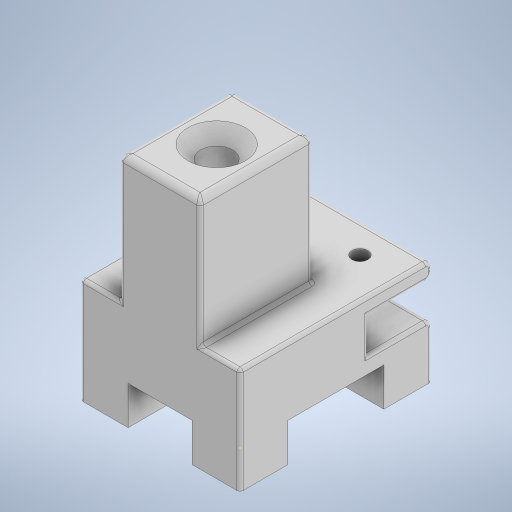
# Autodesk Inventor part: PortaHerramienta1
Saved by Autodesk Inventor 2024 (Build 280153000, 153)
## iProperties
Created: 2023-11-06
Part Number: PortaHerramienta1
Material: Generic
Document SubType Name: Modeling
Designer: Juan_Daleman
Density: 1 g/cm^3
Appearance: Default
Author: Juan_Daleman
Autodesk Inventor part; units mm, degrees
ref_plane "YZ Plane" through (0, 0, 0) normal (1, 0, 0) x (0, 1, 0)
ref_plane "XZ Plane" through (0, 0, 0) normal (0, 1, 0) x (-1, 0, 0)
ref_plane "XY Plane" through (0, 0, 0) normal (0, 0, 1) x (1, 0, 0)
sketch "Sketch1" plane through (0, 0, 0) normal (0, 1, 0) x (-1, 0, 0)
  line L0 (0, 0) -> (50, 0)
  line L1 (50, 0) -> (50, -60)
  line L2 (50, -60) -> (0, -60)
  line L3 (0, -60) -> (0, 0)
  dimension "d0" = 50
  dimension "d1" = 60
  constraints: 8 end point, 2 parallel, 1 horizontal, 1 perpendicular
  measures "d0" distance of L1.end L2.end
  measures "d1" distance of L0.end L1.end
extrude "Extrusion1" add sketch "Sketch1" along normal blind 5
sketch "Sketch2" plane through (0, 5, 0) normal (0, 1, 0) x (1, 0, 0)
  line L0 (-50, 0) -> (0, 0) projected
  line L1 (-50, 60) -> (-50, 0) projected
  line L2 (0, 0) -> (-50, 0)
  line L3 (-50, 0) -> (-50, 40)
  line L4 (-50, 40) -> (0, 40)
  line L5 (0, 40) -> (0, 0)
  dimension "d4" = 40
  constraints: 8 end point, 2 parallel, 1 horizontal, 1 perpendicular, 1 point on line
  measures "d4" distance of L2.end L3.end
extrude "Extrusion2" add sketch "Sketch2" along normal blind 11
sketch "Sketch3" plane through (0, 16, 0) normal (0, 1, 0) x (1, 0, 0)
  line L0 (0, 0) -> (-50, 0)
  line L1 (-50, 0) -> (-50, 60)
  line L2 (-50, 60) -> (0, 60)
  line L3 (0, 60) -> (0, 0)
  constraints: 8 end point, 2 parallel, 1 horizontal, 1 perpendicular
extrude "Extrusion3" add sketch "Sketch3" along normal blind 5
sketch "Sketch4" plane through (0, 21, 0) normal (0, 1, 0) x (1, 0, 0)
  line L0 (0, 0) -> (0, 60) projected
  line L1 (-50, 40) -> (0, 40) projected
  line L2 (0, 60) -> (-50, 60)
  line L3 (-50, 60) -> (-50, 40)
  line L4 (-50, 40) -> (0, 40)
  line L5 (0, 40) -> (0, 60)
  line L6 (-50, 50) -> (0, 50)
  line L7 (-25, 50) -> (-50, 50)
  line L8 (-25, 50) -> (0, 50)
  circle A0 centre (-12.5, 50) radius 2.5
  circle A1 centre (-37.5, 50) radius 2.5
  dimension "d9" = 5
  dimension "d10" = 5
  constraints: 14 end point, 5 midpoint, 2 centre point, 2 collinear, 2 parallel, 1 horizontal, 1 perpendicular
  measures "d9" diameter of A0
  measures "d10" diameter of A1
extrude "Extrusion4" cut sketch "Sketch4" against normal blind 5 contours A0 L6 | L6 A0 | A1 L6 | L6 A1
sketch "Sketch5" plane through (0, 21, 0) normal (0, 1, 0) x (1, 0, 0)
  line L0 (-50, 60) -> (-50, 0) projected
  line L1 (0, 0) -> (-50, 0)
  line L2 (-50, 0) -> (-50, 35)
  line L3 (-50, 35) -> (0, 35)
  line L4 (0, 35) -> (0, 0)
  line L5 (-37.5, 35) -> (-37.5, 0)
  line L6 (-12.5, 35) -> (-12.5, 0)
  dimension "d13" = 35
  constraints: 12 end point, 5 point on line, 3 perpendicular, 2 parallel, 1 horizontal
  measures "d13" distance of L1.end L2.end
extrude "Extrusion5" add sketch "Sketch5" along normal blind 30 contours L3 L6 L1 L5
sketch "Sketch6" plane through (0, 51, 0) normal (0, 1, 0) x (1, 0, 0)
  line L0 (0, 0) -> (0, 60) projected
  line L1 (0, 0) -> (-49.8487, 0)
  line L2 (-49.8487, 0) -> (-49.8487, 35.2322)
  line L3 (-49.8487, 35.2322) -> (0, 35.2322)
  line L4 (0, 35.2322) -> (0, 0)
  line L5 (-49.8487, 17.6161) -> (0, 17.6161) construction
  line L6 (-24.9244, 0) -> (-24.9244, 35.2322) construction
  circle A0 centre (-24.9244, 17.6161) radius 5
  dimension "d16" = 10
  constraints: 12 end point, 5 midpoint, 2 parallel, 1 centre point, 1 horizontal, 1 perpendicular
  measures "d16" diameter of A0
extrude "Extrusion6" cut sketch "Sketch6" against normal blind 30 contours A0
sketch "Sketch7" plane through (0, 51, 0) normal (0, 1, 0) x (1, 0, 0)
  line L0 (-50, 35) -> (-50, 0) projected
  line L1 (0, 0) -> (-50, 0)
  line L2 (-50, 0) -> (-50, 35)
  line L3 (-50, 35) -> (0, 35)
  line L4 (0, 35) -> (0, 0)
  circle A0 centre (-24.9244, 17.6161) radius 5 projected
  circle A1 centre (-24.9244, 17.6161) radius 5
  line L5 (-37.5, 35) -> (-37.5, 0)
  line L6 (-12.5, 35) -> (-12.5, 0)
  constraints: 12 end point, 4 point on line, 2 parallel, 2 perpendicular, 1 centre point, 1 coincident, 1 horizontal
extrude "Extrusion7" add sketch "Sketch7" along normal blind 10 contours L3 L6 L1 L5
chamfer "Chamfer1" distance 4 angle 45 1 edges at (-29.9244, 61, -17.6161)
sketch "Sketch8" plane through (0, 0, 0) normal (0, -1, 0) x (1, 0, 0)
  point P0 (0, 0)
sketch "Sketch9" plane through (0, 0, 0) normal (0, -1, 0) x (1, 0, 0)
  line L0 (0, -60) -> (-50, -60) projected
  line L1 (0, -60) -> (-15, -60)
  line L2 (-15, -60) -> (-15, -45)
  line L3 (-15, -45) -> (0, -45)
  line L4 (0, -45) -> (0, -60)
  line L5 (-50, -60) -> (-50, 0) projected
  line L6 (-50, -60) -> (-35, -60)
  line L7 (-35, -60) -> (-35, -45)
  line L8 (-35, -45) -> (-50, -45)
  line L9 (-50, -45) -> (-50, -60)
  line L10 (0, 0) -> (-15, 0)
  line L11 (-15, 0) -> (-15, -15)
  line L12 (-15, -15) -> (0, -15)
  line L13 (0, -15) -> (0, 0)
  line L14 (-50, 0) -> (-35, 0)
  line L15 (-35, 0) -> (-35, -15)
  line L16 (-35, -15) -> (-50, -15)
  line L17 (-50, -15) -> (-50, 0)
  point P0 (-50, -35)
  dimension "d24" = 15
  dimension "d25" = 15
  dimension "d26" = 15
  dimension "d27" = 15
  dimension "d28" = 15
  dimension "d29" = 15
  constraints: 32 end point, 8 parallel, 4 horizontal, 4 perpendicular, 3 point on line
  measures "d24" distance of L1.end L2.end
  measures "d25" distance of L8.end L7.end
  measures "d26" distance of L7.end L6.end
  measures "d27" distance of L12.end L11.end
  measures "d28" distance of L11.end L10.end
  measures "d29" distance of L15.end L16.end
extrude "Extrusion8" add sketch "Sketch9" along normal blind 12
fillet "Fillet1" radius 2 7 edges at (-25, 61, -35) (-25, 61, 0) (-25, 21, -60) (-25, 16, -60) (-25, 5, -60) (-12.5, 61, -17.5) (-37.5, 61, -17.5)
fillet "Fillet2" radius 1 10 edges at (-50, 20.4142, -59.4142) (-50, 18.5, -60) (-50, 16.5858, -59.4142) (-50, 16, -49) (-50, 21, -29) (0, 20.4142, -59.4142) (0, 18.5, -60) (0, 16.5858, -59.4142) (0, 16, -49) (0, 21, -29)
fillet "Fillet3" radius 1 16 edges at (-49.7071, 20.7071, 0) (-50, 4, 0) (-43.25, 21, 0) (-0.2929, 20.7071, 0) (0, 4, 0) (-6.75, 21, 0) (-50, 4.4142, -59.4142) (-50, 5, -49) (-50, -4.5, -60) (0, 4.4142, -59.4142) (0, 5, -49) (0, -4.5, -60) (0, 16.5, -40) (0, 10.5, -40) (-50, 16.5, -40) (-50, 10.5, -40)
fillet "Fillet4" radius 1 15 edges at (-13.0858, 60.4142, -0.5858) (-12.5, 40, 0) (-12.5, 20.5, 0) (-36.9142, 60.4142, -0.5858) (-37.5, 20.5, 0) (-37.5, 40, 0) (-13.0858, 60.4142, -34.4142) (-12.5, 40, -35) (-36.9142, 60.4142, -34.4142) (-37.5, 40, -35) (-37.5, 20.7071, -0.2929) (-37.5, 21, -18) (-25, 21, -35) (-12.5, 20.7071, -0.2929) (-12.5, 21, -18)
body "Solid1"
